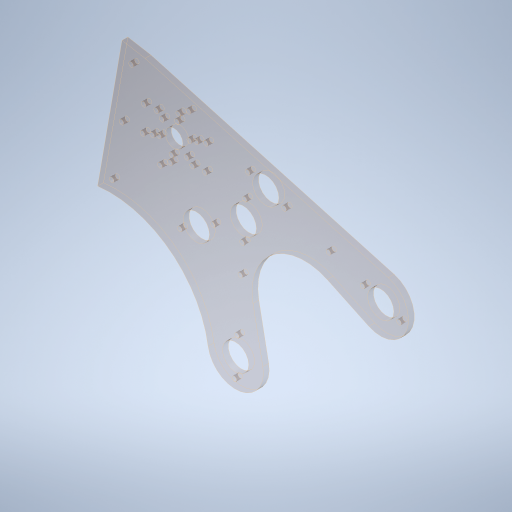
# Autodesk Inventor part: GP7-001
Saved by Autodesk Inventor 2023.4 (Build 274418000, 418)
## iProperties
Created: 2025-02-24
Part Number: GP7-001
Material: Polycarbonate, Smoke
Document SubType Name: Modeling
Designer: dlangdon
Density: 1.2 g/cm^3
Appearance: Polycarbonate - Smoked
Author: dlangdon
Autodesk Inventor part; units mm, degrees
ref_plane "YZ Plane" through (0, 0, 0) normal (1, 0, 0) x (0, 1, 0)
ref_plane "XZ Plane" through (0, 0, 0) normal (0, 1, 0) x (-1, 0, 0)
ref_plane "XY Plane" through (0, 0, 0) normal (0, 0, 1) x (1, 0, 0)
sketch "Sketch1" plane through (0, 0, 0) normal (0, 0, 1) x (1, 0, 0)
  circle A0 centre (78.7027, 64.253) radius 50.8 construction
  circle A1 centre (-78.7027, -64.253) radius 50.8 construction
  circle A2 centre (0, 0) radius 50.8 construction
  line L0 (-39.3513, -32.1265) -> (39.3513, 32.1265) construction
  line L1 (78.7027, 64.253) -> (-78.7027, -64.253) construction
  line L2 (-3.7208, 6.6498) -> (-3.7208, 50.6636) construction
  line L3 (-410.4212, -115.053) -> (454.9708, -115.053) construction
  circle A3 centre (140.9799, -57.903) radius 57.15 construction
  circle A4 centre (78.7027, 64.253) radius 14.2621
  circle A5 centre (-78.7027, -64.253) radius 14.2621
  circle A6 centre (-3.7208, 6.6498) radius 57.15 construction
  circle A7 centre (-78.7027, -64.253) radius 30.1371 construction
  circle A8 centre (78.7027, 64.253) radius 30.1371 construction
  circle A9 centre (-45.946, 108.8074) radius 14.2621
  line L4 (-45.946, 108.8074) -> (78.7027, 64.253) construction
  circle A10 centre (78.7027, 64.253) radius 14.2875 construction
  circle A11 centre (-78.7027, -64.253) radius 14.2875 construction
  circle A12 centre (-70.3302, 67.854) radius 14.2621
  line L5 (-78.7027, -64.253) -> (-70.3302, 67.854) construction
  circle A13 centre (-70.3302, 67.854) radius 23.8316 construction
  circle A14 centre (-45.946, 108.8074) radius 23.8316 construction
  line L6 (20.6869, 58.3256) -> (65.8317, 37.0027)
  line L7 (-49.1354, -58.4201) -> (-59.7901, -4.4114)
  arc A15 (20.6869, 58.3256) -> (-59.7901, -4.4114) centre (-3.7208, 6.6498) ccw
  line L8 (-201.842, 171.7522) -> (-176.8279, 167.3416)
  line L9 (-176.8279, 167.3416) -> (-203.2918, 17.2569) construction
  line L10 (-203.2918, 17.2569) -> (-228.306, 21.6675) construction
  line L11 (-228.306, 21.6675) -> (-201.842, 171.7522) construction
  line L12 (-247.3095, -86.1068) -> (28.2095, -134.6882) construction
  line L13 (-202.9446, 165.4987) -> (190.461, 96.1307) construction
  line L14 (-202.9446, 165.4987) -> (-247.3095, -86.1068) construction
  circle A16 centre (-145.4023, 107.8713) radius 31.75 construction
  line L15 (-71.8375, 44.0702) -> (-75.4896, -13.5547) construction
  circle A17 centre (21.8974, 84.5575) radius 9.525 construction
  line L16 (-189.3349, 169.5469) -> (-215.7989, 19.4622) construction
  line L17 (-192.0916, 153.9131) -> (-213.0422, 35.096) construction
  circle A18 centre (-145.4023, 107.8713) radius 17.4625 construction
  circle A19 centre (-145.4023, 107.8713) radius 9.525
  circle A20 centre (-45.946, 108.8074) radius 30.1816 construction
  line L18 (-201.842, 171.7522) -> (-228.306, 21.6675)
  arc A21 (65.8317, 37.0027) -> (86.8534, 93.267) centre (78.7027, 64.253) ccw
  arc A22 (-108.4816, -68.8852) -> (-49.1354, -58.4201) centre (-78.7027, -64.253) ccw
  line L19 (-145.4023, 107.8713) -> (-128.993, 113.8438) construction
  line L20 (-111.0918, 120.3593) -> (-179.7129, 95.3833) construction
  circle A23 centre (-179.7129, 95.3833) radius 4.7625 construction
  line L21 (0, 0) -> (-3.7208, 6.6498) construction
  circle A24 centre (78.7027, 64.253) radius 28.6512 construction
  line L22 (66.1835, 38.4817) -> (-52.1778, 95.9789) construction
  line L23 (85.3564, 92.1209) -> (-42.6339, 122.6796) construction
  line L24 (-176.8279, 167.3416) -> (86.8534, 93.267)
  line L25 (-145.4023, 107.8713) -> (-121.2929, 36.7784) construction
  circle A25 centre (-121.2929, 36.7784) radius 31.75 construction
  circle A26 centre (-121.2929, 36.7784) radius 14.2621
  line L26 (-70.3302, 67.854) -> (-121.2929, 36.7784) construction
  circle A27 centre (-145.4023, 107.8713) radius 25.4 construction
  arc A28 (-108.4816, -68.8852) -> (-228.306, 21.6675) centre (-215.1488, -85.4777) ccw
  circle A29 centre (-145.4023, 107.8713) radius 36.5125 construction
  line L27 (-178.4939, 123.3021) -> (-145.4023, 107.8713) construction
  point P0 (-73.6635, 15.2577)
  point P1 (-202.5669, 94.5046)
  point P2 (-202.5669, 94.5046)
  point P3 (-142.37, 125.0685)
  point P4 (-158.7794, 119.096)
  point P5 (-161.8117, 101.8988)
  point P6 (-148.4347, 90.6741)
  point P7 (-132.0253, 96.6466)
  point P8 (-121.5341, 116.5586)
  point P9 (-140.9917, 132.8854)
  point P10 (-164.8599, 124.1981)
  point P11 (-169.2705, 99.184)
  point P12 (-149.813, 82.8572)
  point P13 (-125.9448, 91.5445)
  point P14 (-157.8903, 142.1818)
  point P15 (-179.7129, 95.3833)
  point P16 (-132.9143, 73.5608)
  point P17 (-129.9715, 140.9628)
  point P18 (-160.8332, 74.7797)
  point P19 (-112.3108, 92.4404)
  dimension "d7" = 101.6
  dimension "d18" = 47.6631
  dimension "d34" = 34.925
  dimension "d65" = 50.8
  dimension "d3" = 50.772
  dimension "d4" = 0
  dimension "d8" = 101.6
  dimension "d9" = 28.5242
  dimension "d10" = 101.6
  dimension "d11" = 114.3
  dimension "d12" = 114.3
  dimension "d13" = 15.875
  dimension "d14" = 15.875
  dimension "d15" = 132.3721
  dimension "d16" = 28.575
  dimension "d17" = 132.3721
  dimension "d19" = 47.6631
  dimension "d22" = 25.4
  dimension "d23" = 152.4
  dimension "d26" = 255.4869
  dimension "d27" = 63.5
  dimension "d30" = 203.2
  dimension "d31" = 10
  dimension "d32" = 19.05
  dimension "d33" = 120.65
  dimension "d35" = 19.05
  dimension "d36" = 6.35
  dimension "d40" = 360
  dimension "d44" = 9.525
  dimension "d55" = 80
  dimension "d56" = 7.62
  dimension "d58" = 57.3024
  dimension "d59" = 63.5
  dimension "d60" = 75.0697
  dimension "d61" = 59.69
  dimension "d62" = 55
  dimension "d68" = 360
  dimension "d70" = 41.275
  dimension "d71" = 60
  dimension "d82" = 360
  dimension "d87" = 360
  dimension "d89" = 45
  dimension "d90" = 6.35
  dimension "d91" = 20.955
  dimension "d92" = 107.95
  constraints: 56 end point, 26 centre point, 24 coincident, 23 point on circle, 14 tangent, 7 midpoint, 6 equal radius, 5 point on line, 4 collinear, 4 parallel, 2 horizontal, 1 concentric, 1 perpendicular, 1 vertical, 39 other
  measures "d3" angle of L2 L0
  measures "d4" distance between parallel lines of L0 L1
  measures "d8" diameter of A2
  measures "d9" diameter of A4
  measures "d10" diameter of A0
  measures "d11" diameter of A3
  measures "d12" diameter of A6
  measures "d13" radial gap between concentric circles of A5 A7
  measures "d14" radial gap between concentric circles of A4 A8
  measures "d15" distance of L4.start L4.end
  measures "d16" diameter of A10
  measures "d17" distance of L5.start L5.end
  measures "d19" diameter of A14
  measures "d22" distance of L9.end L10.end
  measures "d23" distance of L10.end L8.start
  measures "d26" distance of L13.start L12.start
  measures "d27" diameter of A16
  measures "d30" distance from line of point (0, 0) L9
  measures "d31" angle of L3 L12
  measures "d32" diameter of A17
  measures "d33" distance of L17.start L17.end
  measures "d35" diameter of A19
  measures "d36" radial gap between concentric circles of A14 A20
  measures "d44" diameter of A23
  measures "d55" angle of L1 L21
  measures "d56" distance of L21.start L21.end
  measures "d58" diameter of A24
  measures "d59" diameter of A25
  measures "d60" distance of L19.start L25.end
  measures "d61" distance of L26.start L26.end
  measures "d62" angle of L15 L26
  measures "d70" distance from line of L9 L19.start
  measures "d71" angle of L9 L20
  measures "d89" angle of L20 L27
  measures "d90" distance between parallel lines of L8 L13
  measures "d91" distance from line of L24 L4.start
  measures "d92" radius of A28
extrude "Extrusion1" add sketch "Sketch1" along normal blind 6.35
hole "Hole1" at (21.8974, 84.5575, 0) at (-192.0916, 153.9131, 0) at (-202.5669, 94.5046, 0) at (-213.0422, 35.096, 0) at (-128.993, 113.8438, 0) at (-142.37, 125.0685, 0) at (-158.7794, 119.096, 0) at (-161.8117, 101.8988, 0) at (-148.4347, 90.6741, 0) at (-132.0253, 96.6466, 0) at (-111.0918, 120.3593, 0) at (-179.7129, 95.3833, 0) at (-149.813, 82.8572, 0) at (-169.2705, 99.184, 0) at (-164.8599, 124.1981, 0) at (-140.9917, 132.8854, 0) at (-121.5341, 116.5586, 0) at (-125.9448, 91.5445, 0) at (-73.6635, 15.2577, 0) at (-178.4939, 123.3021, 0) at (-129.9715, 140.9628, 0) at (-112.3108, 92.4404, 0) at (-160.8332, 74.7797, 0) direction (0, 0, 1) diameter 5.1054 end through all clearance for "Flat Head Machine Screw (82)" size "#10" standard "Ansi Unified Screw Threads"
sketch "Sketch2" plane through (0, 0, 6.35) normal (0, 0, 1) x (1, 0, 0)
  circle A0 centre (-125.9448, 91.5445) radius 2.5527 construction
  circle A1 centre (-140.9917, 132.8854) radius 2.5527 construction
  circle A2 centre (-169.2705, 99.184) radius 2.5527 construction
  circle A3 centre (-179.7129, 95.3833) radius 2.5527 construction
  circle A4 centre (-132.0253, 96.6466) radius 2.5527 construction
  circle A5 centre (-161.8117, 101.8988) radius 2.5527 construction
  circle A6 centre (-142.37, 125.0685) radius 2.5527 construction
  circle A7 centre (-213.0422, 35.096) radius 2.5527 construction
  circle A8 centre (-192.0916, 153.9131) radius 2.5527 construction
  circle A9 centre (21.8974, 84.5575) radius 2.5527 construction
  circle A10 centre (-202.5669, 94.5046) radius 2.5527 construction
  circle A11 centre (-128.993, 113.8438) radius 2.5527 construction
  circle A12 centre (-158.7794, 119.096) radius 2.5527 construction
  circle A13 centre (-148.4347, 90.6741) radius 2.5527 construction
  circle A14 centre (-111.0918, 120.3593) radius 2.5527 construction
  circle A15 centre (-149.813, 82.8572) radius 2.5527 construction
  circle A16 centre (-164.8599, 124.1981) radius 2.5527 construction
  circle A17 centre (-121.5341, 116.5586) radius 2.5527 construction
  circle A18 centre (-73.6635, 15.2577) radius 2.5527 construction
  line L0 (-49.1354, -58.4201) -> (-59.7901, -4.4114) construction
  arc A19 (20.6869, 58.3256) -> (-59.7901, -4.4114) centre (-3.7208, 6.6498) ccw construction
  line L1 (20.6869, 58.3256) -> (65.8317, 37.0027) construction
  arc A20 (65.8317, 37.0027) -> (86.8534, 93.267) centre (78.7027, 64.253) ccw construction
  line L2 (86.8534, 93.267) -> (-176.8279, 167.3416) construction
  line L3 (-176.8279, 167.3416) -> (-201.842, 171.7522) construction
  line L4 (-201.842, 171.7522) -> (-228.306, 21.6675) construction
  arc A21 (-108.4816, -68.8852) -> (-228.306, 21.6675) centre (-215.1488, -85.4777) ccw construction
  arc A22 (-108.4816, -68.8852) -> (-49.1354, -58.4201) centre (-78.7027, -64.253) ccw construction
  circle A23 centre (-70.3302, 67.854) radius 14.2621 construction
  circle A24 centre (-145.4023, 107.8713) radius 9.525 construction
  circle A25 centre (-121.2929, 36.7784) radius 14.2621 construction
  circle A26 centre (-45.946, 108.8074) radius 14.2621 construction
  circle A27 centre (-78.7027, -64.253) radius 14.2621 construction
  circle A28 centre (78.7027, 64.253) radius 14.2621 construction
  line L5 (-77.3732, -43.2766) -> (-80.0321, -85.2294) construction
  line L6 (-139.2383, 25.8358) -> (-103.3475, 47.721) construction
  line L7 (-69.0007, 88.8304) -> (-71.6596, 46.8776) construction
  line L8 (-65.7381, 115.8819) -> (-26.1538, 101.7329) construction
  line L9 (58.9105, 71.3275) -> (98.4948, 57.1785) construction
  circle A29 centre (-70.3302, 67.854) radius 14.2621 construction
  line L10 (-45.946, 108.8074) -> (-70.3302, 67.854) construction
  line L11 (-45.946, 108.8074) -> (78.7027, 64.253) construction
  line L12 (-70.3302, 67.854) -> (-121.2929, 36.7784) construction
  line L13 (-70.3302, 67.854) -> (-78.7027, -64.253) construction
  circle A30 centre (-112.3108, 92.4404) radius 2.5527 projected
  point P0 (0, 0)
  point P1 (-116.0598, 70.5176)
  point P2 (-113.1961, 73.3575)
  dimension "d72" = 42.037
  constraints: 19 end point, 14 coincident, 5 collinear, 5 midpoint, 4 equal length, 1 other
  measures "d72" distance of L5.start L5.end
hole "Hole2" at (-77.3732, -43.2766, 6.35) at (-103.3475, 47.721, 6.35) at (-80.0321, -85.2294, 6.35) at (-139.2383, 25.8358, 6.35) at (-71.6596, 46.8776, 6.35) at (-69.0007, 88.8304, 6.35) at (-26.1538, 101.7329, 6.35) at (-65.7381, 115.8819, 6.35) at (98.4948, 57.1785, 6.35) at (58.9105, 71.3275, 6.35) direction (0, 0, -1) diameter 5.1054 end through all clearance for "Flat Head Machine Screw (82)" size "#10" standard "Ansi Unified Screw Threads"
body "Solid1"
